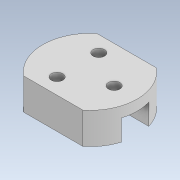
# Autodesk Inventor part: back_hip_cable_protector
Saved by Autodesk Inventor 2020 (Build 240168000, 168)
## iProperties
Created: 2021-02-09
Part Number: back_hip_cable_protector
Material: Generic
Document SubType Name: Modeling
Designer: DELL
Density: 1 g/cm^3
Appearance: Default
Author: DELL
Autodesk Inventor part; units mm, degrees
ref_plane "YZ Plane" through (0, 0, 0) normal (1, 0, 0) x (0, 1, 0)
ref_plane "XZ Plane" through (0, 0, 0) normal (0, 1, 0) x (-1, 0, 0)
ref_plane "XY Plane" through (0, 0, 0) normal (0, 0, 1) x (1, 0, 0)
sketch "Sketch1" plane through (0, 0, 0) normal (0, 1, 0) x (-1, 0, 0)
  circle A0 centre (0, 0) radius 11.5 construction
  line L0 (0, 0) -> (5.75, 9.9593) construction
  line L1 (0, 0) -> (5.75, -9.9593) construction
  line L2 (11.5, 0) -> (0, 0) construction
  circle A1 centre (5.75, 9.9593) radius 1.75
  circle A2 centre (5.75, -9.9593) radius 1.75
  circle A3 centre (0, 0) radius 22.5
  line L3 (14.1421, 17.5) -> (-14.1421, 17.5)
  line L4 (14.1421, -17.5) -> (-14.1421, -17.5)
  line L5 (-22.5, -22.5) -> (22.5, -22.5)
  line L6 (22.5, -22.5) -> (22.5, 22.5)
  line L7 (22.5, 22.5) -> (-22.5, 22.5)
  line L8 (-22.5, 22.5) -> (-22.5, -22.5)
  line L9 (-22.5, -22.5) -> (22.5, 22.5) construction
  line L10 (22.5, -22.5) -> (-22.5, 22.5) construction
  circle A4 centre (-11.5, 0) radius 2.75
  circle A5 centre (5.75, 9.9593) radius 2.75
  circle A6 centre (5.75, -9.9593) radius 2.75
  point P0 (-22.5, 0)
  point P1 (22.5, 0)
  dimension "d0" = 23
  dimension "d1" = 60
  dimension "d2" = 3.5
  dimension "d6" = 35
  dimension "d7" = 45
  dimension "d16" = 5.5
  constraints: 22 end point, 8 point on circle, 7 centre point, 6 coincident, 3 equal radius, 3 horizontal, 3 parallel, 2 midpoint, 2 tangent, 1 perpendicular, 1 point on line, 2 other
  measures "d0" diameter of A0
  measures "d1" angle of L0 L2
  measures "d2" diameter of A1
  measures "d6" distance between parallel lines of L4 L3
  measures "d7" diameter of A3
  measures "d16" diameter of A4
sketch "Sketch2" plane through (0, 0, 0) normal (1, 0, 0) x (0, 1, 0)
  line L0 (0, 17.5) -> (0, 6.5)
  line L1 (0, 6.5) -> (10, 6.5)
  line L2 (10, 6.5) -> (10, -6.5)
  line L3 (10, -6.5) -> (0, -6.5)
  line L4 (0, -6.5) -> (0, -17.5)
  line L5 (11, -17.5) -> (15, -17.5)
  line L6 (15, -17.5) -> (15, 17.5)
  line L7 (15, 17.5) -> (0, 17.5)
  line L8 (11, -17.5) -> (0, -17.5)
  line L9 (0, 0) -> (15, 0) construction
  point P0 (0, -17.5)
  dimension "d5" = 15
  dimension "d14" = 13
  dimension "d15" = 5
  constraints: 20 end point, 6 perpendicular, 2 horizontal, 1 coincident, 1 midpoint, 1 point on line, 1 vertical, 4 other
  measures "d5" distance from line of L9.start L6
  measures "d14" distance between parallel lines of L3 L1
  measures "d15" distance between parallel lines of L6 L2
extrude "Extrusion1" add sketch "Sketch2" along normal mid plane 45
extrude "Extrusion2" cut sketch "Sketch1" along normal through all contours L6 L5 A3 | A3 L7 L6 | L3 A3 | A3 L4 | A3 L8 L7 | L5 L8 A3
extrude "Extrusion3" cut sketch "Sketch1" along normal through all contours A1 | A2
extrude "Extrusion4" cut sketch "Sketch1" along normal through all contours A4
extrude "Extrusion5" cut sketch "Sketch1" against normal blind 8 from surface at 15 contours A1 | A2 | A5 | A6
body "Solid1"
